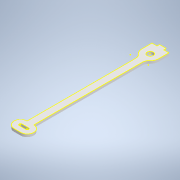
# Autodesk Inventor part: arm
Saved by Autodesk Inventor 2020 (Build 240168000, 168)
## iProperties
Created: 2020-03-11
Part Number: arm
Material: Generic
Document SubType Name: Modeling
Designer: erwin
Density: 1 g/cm^3
Appearance: Default
Author: erwin
Autodesk Inventor part; units mm, degrees
ref_plane "YZ Plane" through (0, 0, 0) normal (1, 0, 0) x (0, 1, 0)
ref_plane "XZ Plane" through (0, 0, 0) normal (0, 1, 0) x (-1, 0, 0)
ref_plane "XY Plane" through (0, 0, 0) normal (0, 0, 1) x (1, 0, 0)
sketch "Sketch1" plane through (0, 0, 0) normal (0, 1, 0) x (-1, 0, 0)
  circle A0 centre (0, 0) radius 30
  line L0 (-12, -45.2841) -> (12, -45.2841)
  line L1 (12, -45.2841) -> (12, -36.2841)
  line L2 (12, -36.2841) -> (-12, -36.2841)
  line L3 (-12, -36.2841) -> (-12, -45.2841)
  line L4 (-12, -45.2841) -> (12, -36.2841) construction
  line L5 (12, -45.2841) -> (-12, -36.2841) construction
  line L6 (12, -36.2841) -> (30, -36.2841)
  line L7 (30, 0) -> (30, -36.2841)
  line L8 (-12, -36.2841) -> (-30, -36.2841)
  line L9 (-30, -36.2841) -> (-30, 0)
  line L10 (-12, 0) -> (12, 0)
  line L11 (12, 0) -> (12, 450)
  line L12 (12, 450) -> (-12, 450)
  line L13 (-12, 450) -> (-12, 0)
  line L14 (12, 450) -> (-12, 450) construction
  line L15 (12, 473.3048) -> (-12, 473.3048)
  line L16 (-12, 426.6952) -> (12, 426.6952)
  arc A1 (12, 426.6952) -> (12, 473.3048) centre (12, 450) ccw
  arc A2 (-12, 473.3048) -> (-12, 426.6952) centre (-12, 450) ccw
  point P0 (0, -40.7841)
  point P1 (0, 450)
  point P2 (-12, 27.4955)
  point P3 (12, 27.4955)
  dimension "d0" = 60
  dimension "d1" = 24
  dimension "d2" = 9
  dimension "d3" = 450
  constraints: 36 end point, 6 equal length, 6 point on circle, 5 tangent, 4 horizontal, 3 centre point, 3 midpoint, 3 perpendicular, 1 coincident, 1 point on line
  measures "d0" diameter of A0
  measures "d1" distance of L2.end L1.end
  measures "d2" distance of L1.end L0.end
  measures "d3" distance of L10.end L11.end
extrude "Extrusion1" add sketch "Sketch1" along normal blind 10
fillet "Fillet1" radius 20 2 edges at (12, 5, 27.4955) (-12, 5, 27.4955)
sketch "Sketch2" plane through (0, 10, 0) normal (0, 1, 0) x (1, 0, 0)
  point P0 (0, 0)
sketch "Sketch3" plane through (0, 10, 0) normal (0, 1, 0) x (1, 0, 0)
  arc A0 (-12, -426.6952) -> (-12, -473.3048) centre (-12, -450) ccw projected
  arc A1 (12, -473.3048) -> (12, -426.6952) centre (12, -450) ccw projected
  point P0 (0, 0)
  constraints: 2 coincident
hole "Hole1" at (-12, 10, 450) at (12, 10, 450) direction (0, -1, 0) diameter 10 end through all
sketch "Sketch4" plane through (0, 10, 0) normal (0, 1, 0) x (1, 0, 0)
  circle A0 centre (-12, -450) radius 5 projected
  circle A1 centre (12, -450) radius 5 projected
  circle A2 centre (12, -450) radius 5 projected
  line L0 (12, -455) -> (-12, -455)
  circle A3 centre (-12, -450) radius 5 projected
  line L1 (-12, -445) -> (12, -445)
  point P0 (0, 0)
  constraints: 4 end point, 2 horizontal, 1 parallel, 1 point on circle, 1 tangent, 1 vertical alignment, 5 other
extrude "Extrusion2" cut sketch "Sketch4" against normal through all contours A0 L1 A1 L0
sketch "Sketch5" plane through (0, 10, 0) normal (0, 1, 0) x (1, 0, 0)
  arc A0 (19.2, -23.0512) -> (30, 0) centre (0, 0) ccw projected
  constraints: 1 coincident
hole "Hole2" at (0, 10, 0) direction (0, -1, 0) diameter 22 end through all
sketch "Sketch6" plane through (0, 10, 0) normal (0, 1, 0) x (1, 0, 0)
  circle A0 centre (0, 0) radius 11 projected
  line L0 (-12, 45.2841) -> (-12, 36.2841) projected
  line L1 (-12, 36.2841) -> (-30, 36.2841) projected
  line L2 (-30, 36.2841) -> (-30, 0) projected
  arc A1 (-30, 0) -> (-19.2, -23.0512) centre (0, 0) ccw projected
  arc A2 (-12, -38.4187) -> (-19.2, -23.0512) centre (-32, -38.4187) ccw projected
  line L3 (-12, -38.4187) -> (-12, -426.6952) projected
  arc A3 (-12, -426.6952) -> (-12, -473.3048) centre (-12, -450) ccw projected
  line L4 (-12, -473.3048) -> (12, -473.3048) projected
  arc A4 (12, -473.3048) -> (12, -426.6952) centre (12, -450) ccw projected
  line L5 (12, -426.6952) -> (12, -38.4187) projected
  arc A5 (19.2, -23.0512) -> (12, -38.4187) centre (32, -38.4187) ccw projected
  arc A6 (19.2, -23.0512) -> (30, 0) centre (0, 0) ccw projected
  line L6 (30, 0) -> (30, 36.2841) projected
  line L7 (30, 36.2841) -> (12, 36.2841) projected
  line L8 (12, 36.2841) -> (12, 45.2841) projected
  line L9 (12, 45.2841) -> (-12, 45.2841) projected
  line L10 (-12, -445) -> (12, -445) projected
  arc A7 (12, -455) -> (12, -445) centre (12, -450) ccw projected
  line L11 (12, -455) -> (-12, -455) projected
  arc A8 (-12, -445) -> (-12, -455) centre (-12, -450) ccw projected
body "Solid1"
